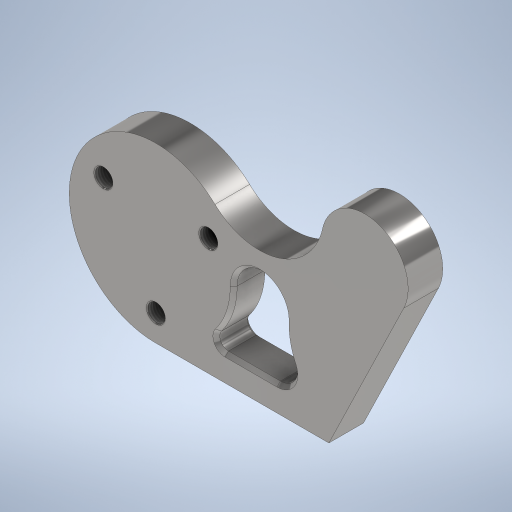
# Autodesk Inventor part: Curve Disc
Saved by Autodesk Inventor 2023 (Build 270158000, 158)
## iProperties
Created: 2023-04-25
Part Number: Curve Disc
Material: Generic
Document SubType Name: Modeling
Designer: dell
Density: 1 g/cm^3
Appearance: Steel - Polished
Author: dell
Autodesk Inventor part; units mm, degrees
ref_plane "YZ Plane" through (0, 0, 0) normal (1, 0, 0) x (0, 1, 0)
ref_plane "XZ Plane" through (0, 0, 0) normal (0, 1, 0) x (-1, 0, 0)
ref_plane "XY Plane" through (0, 0, 0) normal (0, 0, 1) x (1, 0, 0)
sketch "Sketch1" plane through (0, 0, 0) normal (0, 0, 1) x (1, 0, 0)
  arc A0 (-65.8156, 86.4888) -> (-100, 0) centre (-100, 50) ccw
  line L0 (0, 0) -> (-100, 0)
  circle A1 centre (-100, 15) radius 5
  circle A2 centre (-69.6891, 67.5) radius 5
  circle A3 centre (-130.3109, 67.5) radius 5
  arc A4 (-65.8156, 86.4888) -> (-3.6104, 105.5421) centre (-40.1774, 113.8553) ccw
  arc A5 (43.2563, 89.0796) -> (-3.6104, 105.5421) centre (20.7675, 100) ccw
  line L1 (0, 0) -> (43.2563, 89.0796)
  arc A6 (-64, 23) -> (-55, 50) centre (-100, 50) ccw
  arc A7 (-64, 23) -> (-60, 15) centre (-60, 20) ccw
  line L2 (-30, 15) -> (-60, 15)
  arc A8 (-25.0084, 49.4966) -> (-55, 50) centre (-40, 50) ccw
  arc A9 (-30, 15) -> (-20.9152, 29.1794) centre (-30, 25) ccw
  arc A10 (-25.0084, 49.4966) -> (-20.9152, 29.1794) centre (19.9662, 47.9865) ccw
  point P0 (-45, 15)
  dimension "d4" = 100
  dimension "d5" = 10
  dimension "d6" = 35
  dimension "d9" = 360
  dimension "d21" = 15
  dimension "d22" = 25
  dimension "d25" = 5
  dimension "d26" = 50
  dimension "d27" = 37.5
  dimension "d28" = 17.5
  dimension "d29" = 35
  dimension "d30" = 45
  dimension "d32" = 50
  dimension "d52" = 60
  dimension "d55" = 30
  dimension "d56" = 45
  dimension "d57" = 10
  dimension "d58" = 15
  constraints: 16 point on circle, 11 centre point, 10 tangent, 6 end point, 2 horizontal, 1 coincident, 1 midpoint, 1 vertical alignment, 7 other
  measures "d4" distance of L0.end L0.start
  measures "d5" diameter of A1
  measures "d6" distance of A0.centre A1.centre
  measures "d21" distance from line of L0 point (-45, 15)
  measures "d22" radius of A5
  measures "d25" radius of A7
  measures "d26" radius of A0
  measures "d27" radius of A4
  measures "d28" vertical distance of A0.centre A3.centre
  measures "d29" distance of A3.centre A0.centre
  measures "d30" radius of A6
  measures "d32" vertical distance of A0.centre A5.centre
  measures "d52" distance of A0.centre A8.centre
  measures "d55" horizontal distance of A7.centre A9.centre
  measures "d56" radius of A10
  measures "d57" radius of A9
  measures "d58" radius of A8
extrude "Extrusion1" add sketch "Sketch1" along normal blind 20 contours A4 A5 L1 L0 A0 | A6 A8 A10 A9 L2 A7
sketch "Sketch2" plane through (0, 0, 20) normal (0, 0, 1) x (1, 0, 0)
  arc A0 (-25.0084, 49.4966) -> (-55, 50) centre (-40, 50) ccw
  arc A1 (-25.0084, 49.4966) -> (-20.9152, 29.1794) centre (19.9662, 47.9865) ccw
  arc A2 (-64, 23) -> (-60, 15) centre (-60, 20) ccw
  arc A3 (-30, 15) -> (-20.9152, 29.1794) centre (-30, 25) ccw
  line L0 (-100, 0) -> (0, 0) projected
  arc A4 (-64, 23) -> (-55, 50) centre (-100, 50) ccw
  line L1 (-30, 15) -> (-60, 15)
  dimension "d65" = 50
  dimension "d69" = 30
  dimension "d70" = 15
  constraints: 10 point on circle, 5 centre point, 5 tangent, 2 end point, 1 horizontal
  measures "d65" distance from line of L0 A0.centre
  measures "d69" horizontal distance of A2.centre A3.centre
  measures "d70" distance between parallel lines of L0 L1
extrude "Extrusion2" cut sketch "Sketch2" against normal blind 20
chamfer "Chamfer1" distance 2 angle 45 6 edges at (-57.3093, 35.7698, 20) (-39.7483, 64.9979, 20) (-24.1475, 39.0991, 20) (-21.58, 19.6053, 20) (-45, 15, 20) (-64.4721, 17.7639, 20)
chamfer "Chamfer2" distance 2 angle 45 6 edges at (-57.3093, 35.7698, 0) (-64.4721, 17.7639, 0) (-45, 15, 0) (-21.58, 19.6053, 0) (-24.1475, 39.0991, 0) (-39.7483, 64.9979, 0)
chamfer "Chamfer3" distance 0.5 angle 45 3 edges at (-135.3109, 67.5, 0) (-74.6891, 67.5, 0) (-105, 15, 0)
chamfer "Chamfer4" distance 0.5 angle 45 3 edges at (-74.6891, 67.5, 20) (-135.3109, 67.5, 20) (-105, 15, 20)
thread "Thread4" size "M10x1.5" class "6H" standard "ANSI Metric M Profile" full length
thread "Thread5" size "M10x1.5" class "6H" standard "ANSI Metric M Profile" full length
thread "Thread6" size "M10x1.5" class "6H" standard "ANSI Metric M Profile" full length
body "Solid1"
